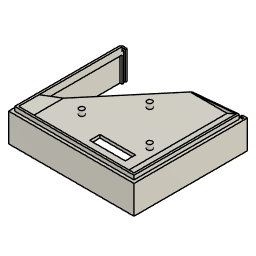
středni kryt (Autodesk Fusion 360 design; units mm, degrees)
Autodesk Fusion 360 part; units mm, degrees
sketch "Sketch1" plane through (0, 0, 0) normal (0, 0, 1) x (1, 0, 0)
  line L0 (0, 0) -> (113.6, 0)
  line L1 (113.6, 0) -> (113.6, 101.8)
  line L2 (113.6, 101.8) -> (0, 101.8)
  line L3 (0, 101.8) -> (0, 0)
  line L4 (-2, -2) -> (115.6, -2)
  line L5 (115.6, -2) -> (115.6, 103.8)
  line L6 (115.6, 103.8) -> (-2, 103.8)
  line L7 (-2, 103.8) -> (-2, -2)
  line L8 (-5, -5) -> (118.6, -5)
  line L9 (118.6, -5) -> (118.6, 106.8)
  line L10 (118.6, 106.8) -> (-5, 106.8)
  line L11 (-5, 106.8) -> (-5, -5)
  dimension "d1" = 113.6
  dimension "d2" = 101.8
  dimension "d3" = 2
  dimension "d4" = 5
  constraint horizontal L0
  constraint vertical L1
  constraint horizontal L2
  constraint vertical L3
  constraint coincident L0.start L3.end
  measures "d1" distance of L0.start L0.end
  measures "d2" distance of L0.start L2.end
extrude "Extrude1" add sketch "Sketch1" along normal blind 3 contours L0 L1 L2 L3
extrude "Extrude2" add sketch "Sketch1" along normal blind 7 contours L4 L5 L6 L7
extrude "Extrude3" add sketch "Sketch1" along normal blind 3 and the other way blind 25 contours L8 L9 L10 L11
sketch "Sketch2" plane through (0, 0, 3) normal (0, 0, 1) x (-1, 0, 0)
  line L0 (0, -101.8) -> (0, 0)
  line L1 (0, 0) -> (-113.6, 0)
  line L2 (-113.6, 0) -> (-113.6, -101.8)
  line L3 (-113.6, -101.8) -> (0, -101.8)
  line L4 (-69, -101.8) -> (0, -20)
  circle A0 centre (-61.3997, -67.6905) radius 2.5
  circle A1 centre (-61.3997, -67.6905) radius 2.5
  circle A2 centre (-96.3997, -32.6905) radius 2.5
  circle A3 centre (-33.8997, -28.1905) radius 2.5
  circle A4 centre (-33.8997, -28.1905) radius 2.5
  circle A5 centre (-96.3997, -32.6905) radius 2.5
  dimension "d15" = 5
  dimension "d16" = 34.1095
  dimension "d17" = 7.6003
  dimension "d18" = 44.6
  dimension "d19" = 20
  dimension "d20" = 5
  dimension "d21" = 5
  dimension "d22" = 17.2003
  dimension "d23" = 69.1095
  dimension "d24" = 33.8997
  dimension "d25" = 28.1905
  constraint coincident L3 L4.start
  constraint coincident L0 L4.end
  measures "d15" diameter of A0
  measures "d16" vertical distance of L4.start A0.centre
  measures "d17" horizontal distance of L4.start A0.centre
  measures "d18" distance of L2.end L4.start
  measures "d19" distance of L4.end L0.end
  measures "d20" diameter of A2
  measures "d21" diameter of A3
  measures "d22" horizontal distance of L2.end A2.centre
  measures "d23" vertical distance of L2.end A2.centre
  measures "d24" horizontal distance of L0.end A3.centre
  measures "d25" vertical distance of L0.end A3.centre
extrude "Extrude4" cut sketch "Sketch2" against normal blind 3 contours L0 L3 L4
extrude "Extrude5" add sketch "Sketch2" along normal blind 5 contours A0 A1 | A2 A5 | A3 A4
sketch "Sketch3" plane through (0, 101.8, 0) normal (0, -1, 0) x (1, 0, 0)
  line L0 (69, 3) -> (113.6, 3)
  line L1 (113.6, 3) -> (113.6, 7)
  line L2 (113.6, 7) -> (0, 7)
  line L3 (0, 7) -> (0, 0)
  line L4 (0, 0) -> (69, 0)
  line L5 (69, 0) -> (69, 3)
  line L6 (69, 3) -> (113.6, 7)
  constraint coincident L0.start L5.end
  constraint coincident L1.end L2.start
extrude "Extrude6" add sketch "Sketch3" along normal blind 1 contours L0 L1 L6
sketch "Sketch4" plane through (0, 0, 3) normal (0, 0, 1) x (-1, 0, 0)
  line L0 (-69, -100.8) -> (-69, -101.8)
  line L1 (-69, -101.8) -> (0, -20)
  line L2 (0, -20) -> (0, 0)
  line L3 (0, 0) -> (-113.6, 0)
  line L4 (-113.6, 0) -> (-113.6, -100.8)
  line L5 (-113.6, -100.8) -> (-69, -100.8)
  circle A0 centre (-96.3997, -32.6905) radius 2.5
  circle A1 centre (-33.8997, -28.1905) radius 2.5
  circle A2 centre (-61.3997, -67.6905) radius 2.5
  line L6 (-95, -20) -> (-60, -20)
  line L7 (-60, -20) -> (-60, -10)
  line L8 (-60, -10) -> (-95, -10)
  line L9 (-95, -10) -> (-95, -20)
  dimension "d34" = 18.6
  dimension "d35" = 10
  dimension "d36" = 35
  dimension "d37" = 10
  constraint horizontal L6
  constraint vertical L7
  constraint horizontal L8
  constraint vertical L9
  measures "d34" horizontal distance of L3.end L8.end
  measures "d35" vertical distance of L3.end L8.end
  measures "d36" distance of L6.start L6.end
  measures "d37" distance of L6.start L8.end
extrude "Extrude7" cut sketch "Sketch4" against normal blind 3 contours L6 L7 L8 L9
extrude "Extrude8" cut 1 faces at (77.4, 106.8, -15.6667) along direction (0, -1, 0) blind 5
extrude "Extrude9" cut 1 faces at (76.4, 103.8, 4.3333) along direction (0, -1, 0) blind 2
chamfer "Chamfer1" distance 2 angle 45 3 edges at (115.6, 49.9, 0) (56.8, -2, 0) (-2, 49.9, 0)
chamfer "Chamfer2" distance 9 distance2 4 1 edges at (113.6, 50.4, 3) measured on face at (91.362, 67.8914, 3)
chamfer "Chamfer3" distance 11 distance2 4 1 edges at (0, 10, 3) measured on face at (88.3626, 67.8914, 3)
sketch "Sketch6" plane through (0, 0, 7) normal (0, 0, 1) x (-1, 0, 0)
  line L0 (0, -101.8) -> (2, -101.8)
  line L1 (2, -101.8) -> (2, 2)
  line L2 (2, 2) -> (-115.6, 2)
  line L3 (-115.6, 2) -> (-115.6, -101.8)
  line L4 (-115.6, -101.8) -> (-113.6, -101.8)
  line L5 (-113.6, -101.8) -> (-113.6, -100.8)
  line L6 (-113.6, -100.8) -> (-113.6, 0)
  line L7 (-113.6, 0) -> (0, 0)
  line L8 (0, 0) -> (0, -20)
  line L9 (0, -20) -> (0, -101.8)
  line L10 (-118.6, -101.8) -> (-113.6, -101.8)
  line L11 (-113.6, -106.8) -> (-118.6, -106.8)
  line L12 (-118.6, -106.8) -> (-118.6, -101.8)
  line L13 (-113.6, -103.5) -> (-116.9, -103.5)
  line L14 (-116.9, -103.5) -> (-116.9, -105.1)
  line L15 (-116.9, -105.1) -> (-113.6, -105.1)
  line L16 (-113.6, -101.8) -> (-113.6, -103.5)
  line L17 (-113.6, -105.1) -> (-113.6, -106.8)
  line L18 (0, -101.8) -> (5, -101.8)
  line L19 (5, -101.8) -> (5, -106.8)
  line L20 (5, -106.8) -> (0, -106.8)
  line L21 (0, -103.5) -> (3.3, -103.5)
  line L22 (3.3, -103.5) -> (3.3, -105.1)
  line L23 (3.3, -105.1) -> (0, -105.1)
  line L24 (0, -106.8) -> (0, -105.1)
  line L25 (0, -103.5) -> (0, -101.8)
  dimension "d49" = 5
  dimension "d50" = 5
  dimension "d51" = 1.6
  dimension "d52" = 1.7
  dimension "d53" = 1.7
  dimension "d54" = 5
  dimension "d55" = 5
  dimension "d56" = 1.6
  dimension "d57" = 1.7
  dimension "d58" = 1.7
  constraint horizontal L10
  constraint vertical L16
  constraint horizontal L11
  constraint vertical L12
  constraint coincident L4.end L5.start
  constraint horizontal L13
  constraint vertical L14
  constraint horizontal L15
  constraint collinear L16 L17
  constraint horizontal L18
  constraint vertical L19
  constraint horizontal L20
  constraint vertical L24
  constraint coincident L0.start L9.end
  constraint horizontal L21
  constraint vertical L22
  constraint horizontal L23
  constraint coincident L21.start L24
  constraint collinear L24 L25
  measures "d49" distance of L10.start L11.end
  measures "d50" distance of L10.start L4.end
  measures "d51" distance of L13.start L15.end
  measures "d52" distance of L10 L13
  measures "d53" distance of L12 L14
  measures "d54" distance of L0.start L18.end
  measures "d55" distance of L0.start L20.end
  measures "d56" distance of L21.start L23.end
  measures "d57" distance of L18 L21
  measures "d58" distance of L19 L22
extrude "Extrude10" add sketch "Sketch6" against normal blind 32 contours L0 L18 L19 L20 L21 L22 L23 L24 L25 | L4 L10 L11 L12 L13 L14 L15 L16 L17
extrude "Extrude11" cut sketch "Sketch6" against normal blind 4 contours L0 L18 L19 L20 L21 L22 L23 L24 L25 | L4 L10 L11 L12 L13 L14 L15 L16 L17
